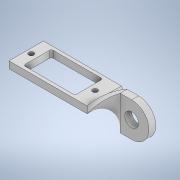
# Autodesk Inventor part: tail
Saved by Autodesk Inventor 2020.3 (Build 243373000, 373)
## iProperties
Created: 2020-08-06
Part Number: tail
Material: Generic
Document SubType Name: Modeling
Designer: aditk
Density: 1 g/cm^3
Appearance: Default
Author: aditk
Autodesk Inventor part; units mm, degrees
ref_plane "YZ Plane" through (0, 0, 0) normal (1, 0, 0) x (0, 1, 0)
ref_plane "XZ Plane" through (0, 0, 0) normal (0, 1, 0) x (-1, 0, 0)
ref_plane "XY Plane" through (0, 0, 0) normal (0, 0, 1) x (1, 0, 0)
sketch "Sketch1" plane through (0, 0, 0) normal (0, 0, 1) x (1, 0, 0)
  circle A0 centre (0, 0) radius 3
  circle A1 centre (0, 0) radius 7.5
  line L0 (0, 7.5) -> (-5, 7.5)
  line L1 (-5, 7.5) -> (-5, -7.5)
  line L2 (-5, -7.5) -> (0, -7.5)
  dimension "d30" = 5
  constraints: 6 end point, 2 centre point, 2 coincident, 2 point on circle, 2 tangent, 1 horizontal, 1 perpendicular
  measures "d30" distance of L0.start L0.end
extrude "Extrusion2" add sketch "Sketch1" along normal blind 3 contours A1 L1 | A1 L1 L0 | L2 L1 A1 picked at (-4.3333, 0)
sketch "Sketch5" plane through (-5, -7.5, 0) normal (-1, 0, 0) x (0, 0, 1)
  line L0 (0, 15) -> (0, 0) projected
  line L1 (0, 0) -> (3, 0) projected
  line L2 (3, 15) -> (3, 0) projected
  line L3 (0, 15) -> (3, 15) projected
  point P0 (0, 7.5)
coil "Coil2" sketch "Sketch5" operation add axis through (-10, 0, 0) along (-1, 0, 0) pitch 40 turns 0.25 hand left
ref_plane "Work Plane2" through (-15, -3, 7.5) normal (0, 1, 0) x (1, 0, 0)
sketch "Sketch6" plane through (-15, -3, 7.5) normal (0, 1, 0) x (1, 0, 0)
  arc A0 (-3.0474, 8.05) -> (-3.0474, 6.95) centre (-4, 7.5) ccw
  line L0 (-1.85, 8.05) -> (-1.85, 12.75)
  line L1 (-1.85, 2.25) -> (-1.85, 6.95)
  line L2 (-7.5, 1.4) -> (-2.7, 1.4)
  line L3 (-33.95, 6.95) -> (-33.95, 2.25)
  line L4 (-33.95, 12.75) -> (-33.95, 8.05)
  arc A1 (-32.7526, 6.95) -> (-32.7526, 8.05) centre (-31.8, 7.5) ccw
  line L5 (-33.95, 6.95) -> (-32.7526, 6.95)
  line L6 (-32.7526, 8.05) -> (-33.95, 8.05)
  line L7 (-28.3, 13.6) -> (-33.1, 13.6)
  line L8 (-2.7, 13.6) -> (-7.5, 13.6)
  arc A2 (-1.85, 12.75) -> (-2.7, 13.6) centre (-2.7, 12.75) ccw
  line L9 (-1.85, 8.05) -> (-3.0474, 8.05)
  line L10 (-3.0474, 6.95) -> (-1.85, 6.95)
  arc A3 (-2.7, 1.4) -> (-1.85, 2.25) centre (-2.7, 2.25) ccw
  arc A4 (-33.95, 2.25) -> (-33.1, 1.4) centre (-33.1, 2.25) ccw
  line L11 (-33.1, 1.4) -> (-28.3, 1.4)
  line L12 (-24.612, 1.4) -> (-28.3, 1.4)
  line L13 (-7.5, 1.4) -> (-21.488, 1.4)
  circle A5 centre (-23.05, 7.5) radius 2.25
  line L14 (-28.3, 13.6) -> (-24.612, 13.6)
  line L15 (-21.488, 13.6) -> (-7.5, 13.6)
  line L16 (-6.65, 2.25) -> (-6.65, 12.75)
  line L17 (-29.15, 12.75) -> (-29.15, 2.25)
  arc A6 (-29.15, 2.25) -> (-28.3, 1.4) centre (-28.3, 2.25) ccw
  arc A7 (-28.3, 13.6) -> (-29.15, 12.75) centre (-28.3, 12.75) ccw
  arc A8 (-33.1, 13.6) -> (-33.95, 12.75) centre (-33.1, 12.75) ccw
  arc A9 (-7.5, 1.4) -> (-6.65, 2.25) centre (-7.5, 2.25) ccw
  arc A10 (-6.65, 12.75) -> (-7.5, 13.6) centre (-7.5, 12.75) ccw
  line L18 (-24.612, 13.6) -> (-21.488, 13.6)
  line L19 (-21.488, 1.4) -> (-24.612, 1.4)
  line L20 (0, 0) -> (0, 15) projected
  line L21 (0, 15) -> (-4, 15)
  line L22 (-4, 15) -> (-4, 0)
  line L23 (-4, 0) -> (0, 0)
  line L24 (-4, 0) -> (-34, 0)
  line L25 (-34, 0) -> (-34, 15)
  line L26 (-34, 15) -> (-4, 15)
  circle A11 centre (-31.8, 7.5) radius 1.1
  circle A12 centre (-4, 7.5) radius 1.1
  point P0 (15, 7.5)
  point P1 (-32.7526, 8.05)
  point P2 (-3.0474, 8.05)
  constraints: 52 end point, 20 point on circle, 11 centre point, 4 perpendicular, 3 horizontal, 2 coincident, 1 midpoint, 1 parallel, 6 other
extrude "Extrusion3" add sketch "Sketch6" along normal blind 3 contours A0 L22 L8 A2 L0 L9 | L9 L0 A2 L8 L22 L21 L20 L23 L2 A3 L1 L10 A12 | A0 L22 L2 A9 L16 A10 L8 | A0 L10 L1 A3 L2 L22 | L8 L15 L18 L14 L7 A8 L4 L6 A11 L5 L3 A4 L11 L12 L19 L13 L2 L22 L24 L25 L26 | A7 L17 A6 L11 A4 L3 L5 A1 L6 L4 A8 L7
body "Solid4"
